Vacuum Attachement (Autodesk Fusion 360 design; units mm, degrees)
Autodesk Fusion 360 part; units mm, degrees
sketch "Sketch1" plane through (0, 0, 0) normal (0, 0, 1) x (1, 0, 0)
  line L0 (0, 0) -> (9.5, 0)
  line L1 (9.5, 0) -> (9.5, 25)
  line L2 (9.5, 25) -> (0, 25)
  line L3 (0, 25) -> (0, 0)
  line L4 (1.25, 25) -> (8.25, 25)
  line L5 (8.25, 25) -> (8.25, 0)
  line L6 (8.25, 0) -> (1.25, 0)
  line L7 (1.25, 0) -> (1.25, 25)
  line L8 (3, 0) -> (0, 6.4335)
  line L9 (3, 0) -> (6, 0) construction
  line L10 (6.5, 0) -> (9.5, 6.4335)
  dimension "d1" = 9.5
  dimension "d2" = 25
  dimension "d3" = 7
  dimension "d4" = 1.25
  dimension "d11" = 3
  dimension "d12" = 3
  dimension "d13" = 65
  dimension "d14" = 65
  constraint horizontal L0
  constraint vertical L1
  constraint horizontal L2
  constraint vertical L3
  constraint coincident L0.start L3.end
  constraint horizontal L4
  constraint vertical L5
  constraint horizontal L6
  constraint vertical L7
  constraint coincident L2 L4.start
  constraint horizontal L9
  constraint coincident L0 L8.start
  constraint coincident L6 L8.start
  constraint coincident L3 L8.end
  constraint coincident L6 L10.start
  constraint coincident L1 L10.end
  measures "d1" distance of L0.start L0.end
  measures "d2" distance of L0.start L2.end
  measures "d3" distance of L4.start L4.end
  measures "d4" distance of L3 L7
  measures "d11" distance of L0.end L10.start
  measures "d12" distance of L0.start L8.start
  measures "d13" angle of L0 L10
  measures "d14" angle of L0 L8
extrude "Extrude1" add sketch "Sketch1" along normal blind 2 contours L2 L3 L7 L8 | L0 L2 L4 L5 L6 L7 L8 L10 | L1 L2 L5 L10
extrude "Extrude2" add sketch "Sketch1" along normal blind 12 contours L0 L2 L4 L5 L6 L7 L8 L10
sketch "Sketch3" plane through (0, 0, 12) normal (0, 0, 1) x (-1, 0, 0)
  line L0 (-3, 0) -> (-6.5, 0)
  line L1 (-6.5, 0) -> (-8.25, -3.7529)
  line L2 (-8.25, -3.7529) -> (-8.25, -25)
  line L3 (-8.25, -25) -> (-1.25, -25)
  line L4 (-1.25, -25) -> (-1.25, -3.7529)
  line L5 (-1.25, -3.7529) -> (-3, 0)
  line L6 (-1.25, -35) -> (-8.25, -35)
  line L7 (-8.25, -35) -> (-8.25, 10)
  line L8 (-8.25, 10) -> (-1.25, 10)
  line L9 (-1.25, 10) -> (-1.25, -35)
  line L10 (-8.25, -35) -> (-1.25, -35)
  line L11 (-1.25, -35) -> (-1.25, -32)
  line L12 (-1.25, -32) -> (-8.25, -32)
  line L13 (-8.25, -32) -> (-8.25, -35)
  line L14 (-1.25, 10) -> (-8.25, 10)
  line L15 (-8.25, 10) -> (-8.25, 7)
  line L16 (-8.25, 7) -> (-1.25, 7)
  line L17 (-1.25, 7) -> (-1.25, 10)
  dimension "d25" = 10
  dimension "d26" = 10
  dimension "d27" = 3
  dimension "d28" = 3
  constraint horizontal L6
  constraint vertical L7
  constraint horizontal L8
  constraint vertical L9
  constraint collinear L2 L7
  constraint collinear L4 L9
  constraint horizontal L10
  constraint vertical L11
  constraint horizontal L12
  constraint vertical L13
  constraint horizontal L14
  constraint vertical L15
  constraint horizontal L16
  constraint vertical L17
  measures "d25" distance of L3 L6
  measures "d26" distance of L0 L8
  measures "d27" distance of L6.end L12.end
  measures "d28" distance of L8.end L16.end
extrude "Extrude3" add sketch "Sketch3" along normal blind 2.5
extrude "Extrude4" add sketch "Sketch3" against normal blind 2 contours L7 L8 L9 L14 L15 L16 L17 | L6 L7 L9 L10 L11 L12 L13
